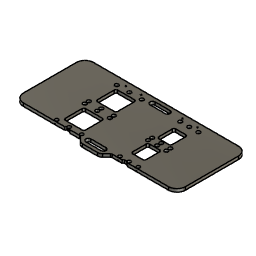
MK2_EU_Baseplate (Autodesk Fusion 360 design; units mm, degrees)
Autodesk Fusion 360 part; units mm, degrees
sketch "Sketch1" plane through (0, 0, 0) normal (0, 0, 1) x (1, 0, 0)
  line L0 (-480, 225) -> (480, 225)
  line L1 (480, 225) -> (480, -225)
  line L2 (480, -225) -> (-480, -225)
  line L3 (-480, -225) -> (-480, 225)
  dimension "d1" = 480
  dimension "d2" = 480
  dimension "d3" = 450
  dimension "d6" = 225
  constraint horizontal L0
  constraint vertical L1
  constraint horizontal L2
  constraint vertical L3
  measures "d1" distance of origin L3
  measures "d2" distance of origin L1
  measures "d3" distance of L0.start L2.end
  measures "d6" distance of origin L0
extrude "Extrude1" add sketch "Sketch1" along normal blind 18
sketch "Sketch2" plane through (0, 0, 18) normal (0, 0, 1) x (-1, 0, 0)
  line L0 (480, 225) -> (-480, 225)
  line L1 (-480, 225) -> (-480, -225)
  line L2 (-480, -225) -> (480, -225)
  line L3 (480, -225) -> (480, 225)
  line L4 (-145, -127.5) -> (-225, -127.5)
  line L5 (-225, -127.5) -> (-225, -27.5)
  line L6 (-225, -27.5) -> (-145, -27.5)
  line L7 (-145, -27.5) -> (-145, -127.5)
  line L8 (-145, 27.5) -> (-225, 27.5)
  line L9 (-225, 27.5) -> (-225, 127.5)
  line L10 (-225, 127.5) -> (-145, 127.5)
  line L11 (-145, 127.5) -> (-145, 27.5)
  line L12 (226.453, -155) -> (106.453, -155)
  line L13 (106.453, -155) -> (106.453, -35)
  line L14 (106.453, -35) -> (226.453, -35)
  line L15 (226.453, -35) -> (226.453, -155)
  line L16 (226.453, -95) -> (106.453, -95) construction
  line L17 (226.453, 35) -> (106.453, 35)
  line L18 (106.453, 35) -> (106.453, 155)
  line L19 (106.453, 155) -> (226.453, 155)
  line L20 (226.453, 155) -> (226.453, 35)
  line L21 (226.453, 95) -> (106.453, 95) construction
  dimension "d7" = 80
  dimension "d8" = 100
  dimension "d9" = 80
  dimension "d11" = 27.5
  dimension "d12" = 27.5
  dimension "d16" = 120
  dimension "d17" = 95
  dimension "d18" = 95
  dimension "d77" = 120
  dimension "d78" = 145
  dimension "d79" = 251.453
  constraint horizontal L4
  constraint vertical L5
  constraint horizontal L6
  constraint vertical L7
  constraint horizontal L8
  constraint vertical L9
  constraint horizontal L10
  constraint vertical L11
  constraint collinear L7 L11
  constraint horizontal L12
  constraint vertical L13
  constraint horizontal L14
  constraint vertical L15
  constraint midpoint L15 L16.start
  constraint midpoint L13 L16.end
  constraint horizontal L17
  constraint vertical L18
  constraint horizontal L19
  constraint vertical L20
  constraint collinear L15 L20
  constraint collinear L13 L18
  constraint midpoint L20 L21.start
  constraint midpoint L18 L21.end
  constraint equal L13 L18
  constraint equal L7 L11
  measures "d7" distance of L4.start L4.end
  measures "d8" distance of L4.start L6.end
  measures "d9" distance of L8.start L8.end
  measures "d11" distance of origin L6
  measures "d12" distance of origin L8
  measures "d16" distance of L12.end L13.end
  measures "d17" distance of origin L16
  measures "d18" distance of origin L21
  measures "d77" distance of L12.start L12.end
  measures "d78" distance of origin L7
  measures "d79" distance of L7 L13
extrude "Extrude2" cut sketch "Sketch2" against normal through all contours L4 L5 L6 L7 | L8 L9 L10 L11 | L12 L13 L14 L15 | L17 L18 L19 L20
sketch "Sketch3" plane through (0, 0, 18) normal (0, 0, 1) x (-1, 0, 0)
  line L0 (-145, 127.5) -> (-145, 27.5)
  line L1 (-145, 27.5) -> (-225, 27.5)
  line L2 (-225, 27.5) -> (-225, 127.5)
  line L3 (-225, 127.5) -> (-145, 127.5)
  line L4 (226.453, 155) -> (226.453, 35)
  line L5 (226.453, 35) -> (106.453, 35)
  line L6 (106.453, 35) -> (106.453, 155)
  line L7 (106.453, 155) -> (226.453, 155)
  line L8 (-145, -27.5) -> (-145, -127.5)
  line L9 (-145, -127.5) -> (-225, -127.5)
  line L10 (-225, -127.5) -> (-225, -27.5)
  line L11 (-225, -27.5) -> (-145, -27.5)
  line L12 (226.453, -35) -> (226.453, -155)
  line L13 (226.453, -155) -> (106.453, -155)
  line L14 (106.453, -155) -> (106.453, -35)
  line L15 (106.453, -35) -> (226.453, -35)
  line L16 (480, 225) -> (-480, 225)
  line L17 (-480, 225) -> (-480, -225)
  line L18 (-480, -225) -> (480, -225)
  line L19 (480, -225) -> (480, 225)
  circle A0 centre (-212, -200) radius 4
  circle A1 centre (-122, -200) radius 4
  circle A2 centre (122, -200) radius 4
  circle A3 centre (212, -200) radius 4
  dimension "d20" = 212
  dimension "d21" = 90
  dimension "d22" = 200
  dimension "d23" = 8
  dimension "d24" = 334
  dimension "d25" = 90
  constraint equal A0 A1
  constraint equal A1 A2
  constraint equal A2 A3
  constraint horizontal A0.centre A2.centre
  constraint horizontal A1.centre A2.centre
  constraint horizontal A2.centre A3.centre
  measures "d20" horizontal distance of origin A0.centre
  measures "d21" distance of A0.centre A1.centre
  measures "d22" vertical distance of origin A0.centre
  measures "d23" diameter of A0
  measures "d24" distance of A0.centre A2.centre
  measures "d25" distance of A2.centre A3.centre
extrude "Extrude3" cut sketch "Sketch3" against normal through all contours A0 | A1 | A2 | A3
sketch "Sketch4" plane through (0, 0, 18) normal (0, 0, 1) x (-1, 0, 0)
  circle A0 centre (122, -200) radius 4
  circle A1 centre (-122, -200) radius 4
  circle A2 centre (212, -200) radius 4
  circle A3 centre (-212, -200) radius 4
  line L0 (480, 225) -> (-480, 225)
  line L1 (-480, 225) -> (-480, -225)
  line L2 (-480, -225) -> (480, -225)
  line L3 (480, -225) -> (480, 225)
  line L4 (-1.75, 0) -> (-22.5, 0)
  circle A4 centre (122, -200) radius 4
  circle A5 centre (-122, -200) radius 4
  circle A6 centre (212, -200) radius 4
  circle A7 centre (-212, -200) radius 4
  line L5 (226.453, 35) -> (226.453, 155)
  line L6 (226.453, 155) -> (106.453, 155)
  line L7 (106.453, 155) -> (106.453, 35)
  line L8 (106.453, 35) -> (226.453, 35)
  line L9 (226.453, -155) -> (226.453, -35)
  line L10 (226.453, -35) -> (106.453, -35)
  line L11 (106.453, -35) -> (106.453, -155)
  line L12 (106.453, -155) -> (226.453, -155)
  line L13 (-480, 225) -> (480, 225)
  line L14 (480, 225) -> (480, -225)
  line L15 (480, -225) -> (-480, -225)
  line L16 (-480, -225) -> (-480, 225)
  circle A8 centre (122, -200) radius 4
  circle A9 centre (-122, -200) radius 4
  circle A10 centre (212, -200) radius 4
  circle A11 centre (-212, -200) radius 4
  line L17 (-145, 127.5) -> (-145, 27.5)
  line L18 (-145, 27.5) -> (-225, 27.5)
  line L19 (-225, 27.5) -> (-225, 127.5)
  line L20 (-225, 127.5) -> (-145, 127.5)
  line L21 (226.453, 155) -> (226.453, 35)
  line L22 (226.453, 35) -> (106.453, 35)
  line L23 (106.453, 35) -> (106.453, 155)
  line L24 (106.453, 155) -> (226.453, 155)
  line L25 (-145, -27.5) -> (-145, -127.5)
  line L26 (-145, -127.5) -> (-225, -127.5)
  line L27 (-225, -127.5) -> (-225, -27.5)
  line L28 (-225, -27.5) -> (-145, -27.5)
  line L29 (226.453, -35) -> (226.453, -155)
  line L30 (226.453, -155) -> (106.453, -155)
  line L31 (106.453, -155) -> (106.453, -35)
  line L32 (106.453, -35) -> (226.453, -35)
  line L33 (480, 225) -> (-480, 225)
  line L34 (-480, 225) -> (-480, -225)
  line L35 (-480, -225) -> (480, -225)
  line L36 (480, -225) -> (480, 225)
  point P0 (96, -178)
  point P1 (170, -178)
  point P2 (244, -178)
  point P3 (96, -12)
  point P4 (170, -12)
  point P5 (244, -12)
  point P6 (-239, -178)
  point P7 (-185, -178)
  point P8 (-131, -178)
  point P9 (-131, -12)
  point P10 (-185, -12)
  point P11 (-239, -12)
  point P12 (96, 178)
  point P13 (170, 178)
  point P14 (244, 178)
  point P15 (244, 12)
  point P16 (170, 12)
  point P17 (96, 12)
  point P18 (-239, 178)
  point P19 (-185, 178)
  point P20 (-131, 178)
  point P21 (-131, 12)
  point P22 (-185, 12)
  point P23 (-239, 12)
  dimension "d27" = 74
  dimension "d28" = 74
  dimension "d29" = 166
  dimension "d32" = 54
  dimension "d33" = 54
  dimension "d80" = 17.547
  dimension "d82" = 23
  dimension "d93" = 14
  constraint vertical P0 P3
  constraint vertical P1 P4
  constraint vertical P2 P5
  constraint horizontal P3 P4
  constraint horizontal P4 P5
  constraint horizontal P0 P1
  constraint horizontal P1 P2
  constraint vertical P6 P11
  constraint vertical P7 P10
  constraint vertical P8 P9
  constraint horizontal P6 P7
  constraint horizontal P7 P8
  constraint horizontal P10 P11
  constraint horizontal P9 P10
  constraint horizontal P5 P11
  constraint horizontal P2 P6
  constraint symmetric P0 L4 P12
  constraint symmetric P1 L4 P13
  constraint symmetric P2 L4 P14
  constraint symmetric P3 L4 P17
  constraint symmetric P4 L4 P16
  constraint symmetric P5 L4 P15
  constraint symmetric P6 L4 P18
  constraint symmetric P7 L4 P19
  constraint symmetric P8 L4 P20
  constraint symmetric P9 L4 P21
  constraint symmetric P10 L4 P22
  constraint symmetric P11 L4 P23
  measures "d27" distance of P0 P1
  measures "d28" distance of P1 P2
  measures "d29" vertical distance of P0 P3
  measures "d32" distance of P6 P7
  measures "d33" distance of P7 P8
  measures "d80" distance of P2 L9
  measures "d82" distance of P2 L12
  measures "d93" distance of P8 L25
hole "Hole5" at (131, -178, 18) at (185, -178, 18) at (239, -178, 18) at (-96, -178, 18) at (-170, -178, 18) at (-244, -178, 18) direction (0, 0, -1) diameter 8 depth 18 tip angle 118 counterbore diameter 20 counterbore depth 13
hole "Hole6" at (-244, 12, 18) at (-170, 12, 18) at (-96, 12, 18) at (-96, -12, 18) at (-170, -12, 18) at (-244, -12, 18) at (131, 12, 18) at (185, 12, 18) at (185, -12, 18) at (131, -12, 18) at (239, -12, 18) at (239, 12, 18) at (-244, 178, 18) at (-170, 178, 18) at (-96, 178, 18) at (131, 178, 18) at (185, 178, 18) at (239, 178, 18) direction (0, 0, -1) diameter 9 depth 18 tip angle 118 counterbore diameter 22 counterbore depth 13
sketch "Sketch5" plane through (0, 0, 18) normal (0, 0, 1) x (-1, 0, 0)
  circle A0 centre (122, -200) radius 4
  circle A1 centre (-122, -200) radius 4
  circle A2 centre (212, -200) radius 4
  circle A3 centre (-212, -200) radius 4
  line L0 (-145, 127.5) -> (-145, 27.5)
  line L1 (-145, 27.5) -> (-225, 27.5)
  line L2 (-225, 27.5) -> (-225, 127.5)
  line L3 (-225, 127.5) -> (-145, 127.5)
  line L4 (226.453, 155) -> (226.453, 35)
  line L5 (226.453, 35) -> (106.453, 35)
  line L6 (106.453, 35) -> (106.453, 155)
  line L7 (106.453, 155) -> (226.453, 155)
  line L8 (-145, -27.5) -> (-145, -127.5)
  line L9 (-145, -127.5) -> (-225, -127.5)
  line L10 (-225, -127.5) -> (-225, -27.5)
  line L11 (-225, -27.5) -> (-145, -27.5)
  line L12 (226.453, -35) -> (226.453, -155)
  line L13 (226.453, -155) -> (106.453, -155)
  line L14 (106.453, -155) -> (106.453, -35)
  line L15 (106.453, -35) -> (226.453, -35)
  line L16 (480, 225) -> (-480, 225)
  line L17 (-480, 225) -> (-480, -225)
  line L18 (-480, -225) -> (480, -225)
  line L19 (480, -225) -> (480, 225)
  line L20 (45, 205) -> (-45, 205)
  arc A4 (-45, 205) -> (-45, 175) centre (-45, 190) ccw
  line L21 (-45, 175) -> (45, 175)
  arc A5 (45, 175) -> (45, 205) centre (45, 190) ccw
  line L22 (45, 190) -> (-45, 190) construction
  line L23 (-1.75, 0) -> (-22.5, 0)
  line L24 (45, -190) -> (-45, -190) construction
  line L25 (-45, -175) -> (45, -175)
  arc A6 (-45, -175) -> (-45, -205) centre (-45, -190) ccw
  line L26 (45, -205) -> (-45, -205)
  arc A7 (45, -205) -> (45, -175) centre (45, -190) ccw
  circle A8 centre (-239, 12) radius 11
  circle A9 centre (-185, 12) radius 11
  circle A10 centre (-131, -12) radius 11
  circle A11 centre (170, 12) radius 11
  circle A12 centre (96, -12) radius 11
  circle A13 centre (244, -12) radius 11
  circle A14 centre (170, -12) radius 11
  circle A15 centre (96, 12) radius 11
  circle A16 centre (244, 12) radius 11
  circle A17 centre (-185, -12) radius 11
  circle A18 centre (-131, 12) radius 11
  circle A19 centre (-239, -12) radius 11
  circle A20 centre (170, 178) radius 10
  circle A21 centre (-239, 178) radius 10
  circle A22 centre (-131, 178) radius 10
  circle A23 centre (-185, 178) radius 10
  circle A24 centre (96, 178) radius 10
  circle A25 centre (244, 178) radius 10
  circle A26 centre (-185, -178) radius 11
  circle A27 centre (96, -178) radius 11
  circle A28 centre (244, -178) radius 11
  circle A29 centre (170, -178) radius 11
  circle A30 centre (-131, -178) radius 11
  circle A31 centre (-239, -178) radius 11
  dimension "d39" = 30
  dimension "d40" = 90
  dimension "d41" = 45
  dimension "d42" = 190
  constraint tangent L20 A4
  constraint tangent A4 L21
  constraint parallel L20 L21
  constraint tangent L21 A5
  constraint tangent L20 A5
  constraint perpendicular L10 L22
  constraint symmetric L20.start L23 L26.start
  constraint symmetric L20.end L23 A6.end
  constraint symmetric A4.end L23 L25.start
  constraint symmetric L21.end L23 L25.end
  constraint symmetric A4 L23 A6
  constraint symmetric A5 L23 A7
  measures "d39" distance of L20 L21
  measures "d40" distance of L20.start L20.end
  measures "d41" horizontal distance of origin A4.centre
  measures "d42" distance of origin L22
extrude "Extrude4" cut sketch "Sketch5" against normal through all contours L20 A4 L21 A5 | L25 A6 L26 A7
sketch "Sketch6" plane through (0, 0, 18) normal (0, 0, 1) x (-1, 0, 0)
  line L0 (-45, -175) -> (45, -175)
  arc A0 (45, -205) -> (45, -175) centre (45, -190) ccw
  line L1 (45, -205) -> (-45, -205)
  arc A1 (-45, -175) -> (-45, -205) centre (-45, -190) ccw
  line L2 (45, 175) -> (-45, 175)
  arc A2 (-45, 205) -> (-45, 175) centre (-45, 190) ccw
  line L3 (-45, 205) -> (45, 205)
  arc A3 (45, 175) -> (45, 205) centre (45, 190) ccw
  circle A4 centre (122, -200) radius 4
  circle A5 centre (-122, -200) radius 4
  circle A6 centre (212, -200) radius 4
  circle A7 centre (-212, -200) radius 4
  line L4 (-145, 127.5) -> (-145, 27.5)
  line L5 (-145, 27.5) -> (-225, 27.5)
  line L6 (-225, 27.5) -> (-225, 127.5)
  line L7 (-225, 127.5) -> (-145, 127.5)
  line L8 (226.453, 155) -> (226.453, 35)
  line L9 (226.453, 35) -> (106.453, 35)
  line L10 (106.453, 35) -> (106.453, 155)
  line L11 (106.453, 155) -> (226.453, 155)
  line L12 (-145, -27.5) -> (-145, -127.5)
  line L13 (-145, -127.5) -> (-225, -127.5)
  line L14 (-225, -127.5) -> (-225, -27.5)
  line L15 (-225, -27.5) -> (-145, -27.5)
  line L16 (226.453, -35) -> (226.453, -155)
  line L17 (226.453, -155) -> (106.453, -155)
  line L18 (106.453, -155) -> (106.453, -35)
  line L19 (106.453, -35) -> (226.453, -35)
  line L20 (480, 225) -> (-480, 225)
  line L21 (-480, 225) -> (-480, -225)
  line L22 (-480, -225) -> (480, -225)
  line L23 (480, -225) -> (480, 225)
  line L24 (480, 190) -> (92, 190)
  line L25 (92, 190) -> (57, 225)
  line L26 (-57, 225) -> (-92, 190)
  line L27 (-92, 190) -> (-480, 190)
  circle A8 centre (-239, 12) radius 11
  circle A9 centre (-185, 12) radius 11
  circle A10 centre (-131, -12) radius 11
  circle A11 centre (170, 12) radius 11
  circle A12 centre (96, -12) radius 11
  circle A13 centre (244, -12) radius 11
  circle A14 centre (170, -12) radius 11
  circle A15 centre (96, 12) radius 11
  circle A16 centre (244, 12) radius 11
  circle A17 centre (-185, -12) radius 11
  circle A18 centre (-131, 12) radius 11
  circle A19 centre (-239, -12) radius 11
  circle A20 centre (170, 178) radius 10
  circle A21 centre (-239, 178) radius 10
  circle A22 centre (-131, 178) radius 10
  circle A23 centre (-185, 178) radius 10
  circle A24 centre (96, 178) radius 10
  circle A25 centre (244, 178) radius 10
  circle A26 centre (-185, -178) radius 11
  circle A27 centre (96, -178) radius 11
  circle A28 centre (244, -178) radius 11
  circle A29 centre (170, -178) radius 11
  circle A30 centre (-131, -178) radius 11
  circle A31 centre (-239, -178) radius 11
  dimension "d44" = 35
  dimension "d45" = 135
  dimension "d46" = 57
  dimension "d47" = 57
  dimension "d48" = 135
  constraint coincident L23 L24.start
  constraint perpendicular L23 L24
  constraint coincident L20 L25.end
  constraint coincident L20 L26.start
  constraint coincident L21 L27.end
  constraint perpendicular L21 L27
  constraint collinear L24 L27
  measures "d44" distance of L20 L24
  measures "d45" angle of L24 L25
  measures "d46" horizontal distance of origin L25.end
  measures "d47" horizontal distance of origin L26.start
  measures "d48" angle of L26 L27
extrude "Extrude5" cut sketch "Sketch6" against normal through all contours L20 L23 L24 L25 | L20 L21 L26 L27
fillet "Fillet1" radius 30 2 edges at (-57, -225, 9) (57, -225, 9)
fillet "Fillet1" radius 10 18 edges at (-92, -190, 9) (92, -190, 9) (-106.453, 155, 9) (-106.453, -35, 9) (225, 127.5, 9) (225, -27.5, 9) (-226.453, 155, 9) (145, 127.5, 9) (145, -27.5, 9) (-226.453, -35, 9) (-106.453, -155, 9) (225, -127.5, 9) (-226.453, -155, 9) (145, -127.5, 9) (-226.453, 35, 9) (145, 27.5, 9) (-106.453, 35, 9) (225, 27.5, 9)
fillet "Fillet1" radius 50 4 edges at (480, -190, 9) (-480, -190, 9) (-480, 225, 9) (480, 225, 9)
sketch "Sketch7" plane through (0, 0, 0) normal (0, 0, -1) x (1, 0, 0)
  arc A0 (430, -225) -> (480, -175) centre (430, -175) ccw
  line L0 (480, -175) -> (480, 140)
  arc A1 (480, 140) -> (430, 190) centre (430, 140) ccw
  line L1 (430, 190) -> (96.1421, 190)
  arc A2 (89.0711, 192.9289) -> (96.1421, 190) centre (96.1421, 200) ccw
  line L2 (89.0711, 192.9289) -> (65.7868, 216.2132)
  arc A3 (65.7868, 216.2132) -> (44.5736, 225) centre (44.5736, 195) ccw
  line L3 (44.5736, 225) -> (-44.5736, 225)
  arc A4 (-44.5736, 225) -> (-65.7868, 216.2132) centre (-44.5736, 195) ccw
  line L4 (-65.7868, 216.2132) -> (-89.0711, 192.9289)
  arc A5 (-96.1421, 190) -> (-89.0711, 192.9289) centre (-96.1421, 200) ccw
  line L5 (-96.1421, 190) -> (-430, 190)
  arc A6 (-430, 190) -> (-480, 140) centre (-430, 140) ccw
  line L6 (-480, 140) -> (-480, -175)
  arc A7 (-480, -175) -> (-430, -225) centre (-430, -175) ccw
  line L7 (-430, -225) -> (430, -225)
  line L8 (-226.453, -145) -> (-226.453, -45)
  arc A8 (-216.453, -35) -> (-226.453, -45) centre (-216.453, -45) ccw
  line L9 (-216.453, -35) -> (-116.453, -35)
  arc A9 (-106.453, -45) -> (-116.453, -35) centre (-116.453, -45) ccw
  line L10 (-106.453, -45) -> (-106.453, -145)
  arc A10 (-116.453, -155) -> (-106.453, -145) centre (-116.453, -145) ccw
  line L11 (-116.453, -155) -> (-216.453, -155)
  arc A11 (-226.453, -145) -> (-216.453, -155) centre (-216.453, -145) ccw
  line L12 (145, -117.5) -> (145, -37.5)
  arc A12 (155, -27.5) -> (145, -37.5) centre (155, -37.5) ccw
  line L13 (155, -27.5) -> (215, -27.5)
  arc A13 (225, -37.5) -> (215, -27.5) centre (215, -37.5) ccw
  line L14 (225, -37.5) -> (225, -117.5)
  arc A14 (215, -127.5) -> (225, -117.5) centre (215, -117.5) ccw
  line L15 (215, -127.5) -> (155, -127.5)
  arc A15 (145, -117.5) -> (155, -127.5) centre (155, -117.5) ccw
  line L16 (-226.453, 45) -> (-226.453, 145)
  arc A16 (-216.453, 155) -> (-226.453, 145) centre (-216.453, 145) ccw
  line L17 (-216.453, 155) -> (-116.453, 155)
  arc A17 (-106.453, 145) -> (-116.453, 155) centre (-116.453, 145) ccw
  line L18 (-106.453, 145) -> (-106.453, 45)
  arc A18 (-116.453, 35) -> (-106.453, 45) centre (-116.453, 45) ccw
  line L19 (-116.453, 35) -> (-216.453, 35)
  arc A19 (-226.453, 45) -> (-216.453, 35) centre (-216.453, 45) ccw
  line L20 (145, 37.5) -> (145, 117.5)
  arc A20 (155, 127.5) -> (145, 117.5) centre (155, 117.5) ccw
  line L21 (155, 127.5) -> (215, 127.5)
  arc A21 (225, 117.5) -> (215, 127.5) centre (215, 117.5) ccw
  line L22 (225, 117.5) -> (225, 37.5)
  arc A22 (215, 27.5) -> (225, 37.5) centre (215, 37.5) ccw
  line L23 (215, 27.5) -> (155, 27.5)
  arc A23 (145, 37.5) -> (155, 27.5) centre (155, 37.5) ccw
  circle A24 centre (212, -200) radius 4
  circle A25 centre (-212, -200) radius 4
  circle A26 centre (122, -200) radius 4
  circle A27 centre (-122, -200) radius 4
  line L24 (45, 175) -> (-45, 175)
  arc A28 (-45, 205) -> (-45, 175) centre (-45, 190) ccw
  line L25 (-45, 205) -> (45, 205)
  arc A29 (45, 175) -> (45, 205) centre (45, 190) ccw
  line L26 (-45, -175) -> (45, -175)
  arc A30 (45, -205) -> (45, -175) centre (45, -190) ccw
  line L27 (45, -205) -> (-45, -205)
  arc A31 (-45, -175) -> (-45, -205) centre (-45, -190) ccw
  line L28 (177.5, 197) -> (162.5, 197)
  arc A32 (162.5, 197) -> (162.5, 183) centre (162.5, 190) ccw
  line L29 (162.5, 183) -> (177.5, 183)
  arc A33 (177.5, 183) -> (177.5, 197) centre (177.5, 190) ccw
  line L30 (177.5, 190) -> (162.5, 190) construction
  line L31 (-162.5, 197) -> (-177.5, 197)
  arc A34 (-177.5, 197) -> (-177.5, 183) centre (-177.5, 190) ccw
  line L32 (-177.5, 183) -> (-162.5, 183)
  arc A35 (-162.5, 183) -> (-162.5, 197) centre (-162.5, 190) ccw
  line L33 (-162.5, 190) -> (-177.5, 190) construction
  circle A36 centre (-244, 178) radius 4
  circle A37 centre (-96, 178) radius 4
  circle A38 centre (185, 178) radius 4
  circle A39 centre (131, 178) radius 4
  circle A40 centre (239, 178) radius 4
  circle A41 centre (-170, 178) radius 4
  circle A42 centre (239, -12) radius 4.5
  circle A43 centre (131, 12) radius 4.5
  circle A44 centre (185, -12) radius 4.5
  circle A45 centre (-244, 12) radius 4.5
  circle A46 centre (-96, 12) radius 4.5
  circle A47 centre (-170, -12) radius 4.5
  circle A48 centre (-244, -12) radius 4.5
  circle A49 centre (-96, -12) radius 4.5
  circle A50 centre (-170, 12) radius 4.5
  circle A51 centre (131, -12) radius 4.5
  circle A52 centre (185, 12) radius 4.5
  circle A53 centre (239, 12) radius 4.5
  circle A54 centre (239, -178) radius 4.5
  circle A55 centre (131, -178) radius 4.5
  circle A56 centre (-170, -178) radius 4.5
  circle A57 centre (-244, -178) radius 4.5
  circle A58 centre (-96, -178) radius 4.5
  circle A59 centre (185, -178) radius 4.5
  point P0 (170, 190)
  point P1 (-170, 190)
  dimension "d56" = 7.5
  dimension "d57" = 14
  dimension "d58" = 14
  dimension "d60" = 15
  constraint tangent L28 A32
  constraint tangent A32 L29
  constraint parallel L28 L29
  constraint tangent L29 A33
  constraint tangent L28 A33
  constraint parallel L1 L30
  constraint coincident L1 P0
  constraint midpoint L30 P0
  constraint tangent L31 A34
  constraint tangent A34 L32
  constraint parallel L31 L32
  constraint tangent L32 A35
  constraint tangent L31 A35
  constraint parallel L5 L33
  constraint coincident L5 P1
  constraint midpoint L33 P1
  measures "d56" distance of A32.centre P0
  measures "d57" diameter of A32
  measures "d58" distance of L31 L32
  measures "d60" distance of A35.centre A34.centre
extrude "Extrude6" cut sketch "Sketch7" against normal through all contours L1 A32 L29 A33 | L5 A34 L32 A35
equation "d6 = d3 / 2"
equation "d12 = d11"
equation "d18 = d17"
equation "d25 = d21"
equation "d28 = d27"
equation "d33 = d32"
equation "d41 = d40 / 2"
equation "d47 = d46"
equation "d78 = 150 mm - 5 mm"
equation "d79 = 256.453 mm - 5 mm"
